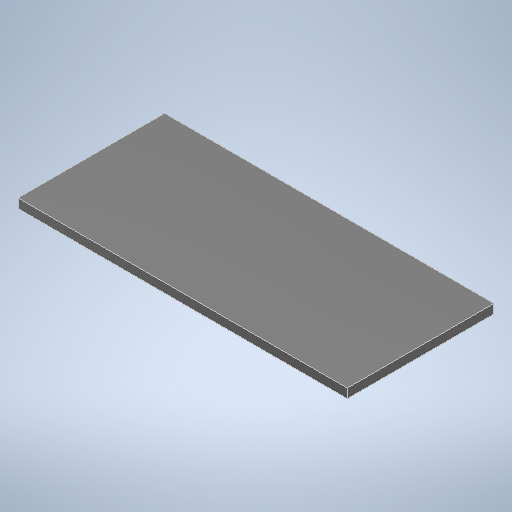
# Autodesk Inventor part: Top Insulation 0p5in
Saved by Autodesk Inventor 2025 (Build 290162000, 162)
## iProperties
Created: 2025-06-12
Part Number: Top Insulation 0p5in
Material: Thermoplastic Resin
Document SubType Name: Modeling
Designer: Caleb Fangmeier
Density: 1.28 g/cm^3
Appearance: Smooth - Black
Author: Caleb Fangmeier
Autodesk Inventor part; units mm, degrees
ref_plane "YZ Plane" through (0, 0, 0) normal (1, 0, 0) x (0, 1, 0)
ref_plane "XZ Plane" through (0, 0, 0) normal (0, 1, 0) x (-1, 0, 0)
ref_plane "XY Plane" through (0, 0, 0) normal (0, 0, 1) x (1, 0, 0)
sketch "Sketch1" plane through (0, 0, 0) normal (0, 1, 0) x (-1, 0, 0)
  line L0 (-228, 101.5) -> (228, 101.5)
  line L1 (228, 101.5) -> (228, -101.5)
  line L2 (228, -101.5) -> (-228, -101.5)
  line L3 (-228, -101.5) -> (-228, 101.5)
  line L4 (-228, 101.5) -> (228, -101.5) construction
  line L5 (228, 101.5) -> (-228, -101.5) construction
  point P0 (0, 0)
  dimension "d0" = 203
  dimension "d1" = 456
  constraints: 12 end point, 2 midpoint, 2 parallel, 1 horizontal, 1 perpendicular
  measures "d0" distance of L0.end L1.end
  measures "d1" distance of L1.end L2.end
extrude "Extrusion1" add sketch "Sketch1" along normal blind 12.7
body "Solid1"
